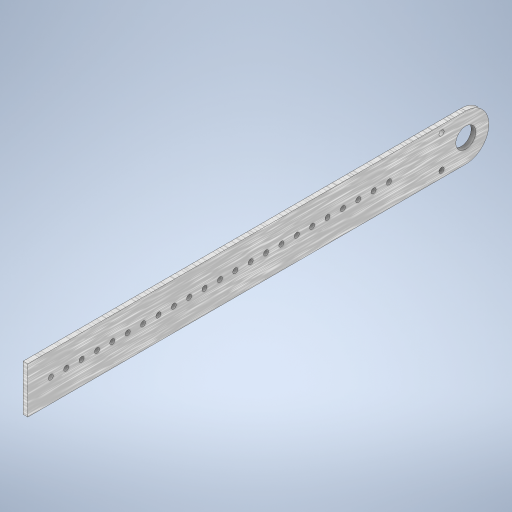
# Autodesk Inventor part: shoulder1_plate_top
Saved by Autodesk Inventor 2024 (Build 280153000, 153)
## iProperties
Company: 細田研究室
Created: 2025-06-07
Part Number: shoulder1_plate_top
Material: アルミニウム 5052
Document SubType Name: Modeling
Designer: HosodaLab2
Density: 2.68 g/cm^3
Appearance: サテン - ブラシ仕上げ 重厚
Mass: 70.367 g
Surface Area: 200.69 cm^2
Volume: 26.0618 cm^3
Stock Number: 1
個数: 1
Author: HosodaLab2
Autodesk Inventor part; units mm, degrees
ref_plane "YZ Plane" through (0, 0, 0) normal (1, 0, 0) x (0, 1, 0)
ref_plane "XZ Plane" through (0, 0, 0) normal (0, 1, 0) x (-1, 0, 0)
ref_plane "XY Plane" through (0, 0, 0) normal (0, 0, 1) x (1, 0, 0)
sketch "スケッチ1" plane through (0, 0, 0) normal (0, 1, 0) x (-1, 0, 0)
  line L0 (0, 0) -> (-300, 0)
  line L1 (-300, 0) -> (-300, -30)
  line L2 (-300, -30) -> (0, -30)
  line L3 (0, -30) -> (0, 0)
  arc A0 (-15, -30) -> (-15, 0) centre (-15, -15) ccw
  point P0 (-15, -15)
  dimension "d0" = 300
  dimension "d1" = 30
  dimension "d2" = 15
  dimension "d3" = 15
  dimension "d43" = 15
  constraints: 8 end point, 2 parallel, 2 point on circle, 2 point on line, 2 tangent, 1 centre point, 1 horizontal, 1 perpendicular
  measures "d0" distance of L2.end L1.end
  measures "d1" distance of L1.end L0.end
  measures "d2" distance from line of L2 point (-15, -15)
  measures "d3" distance from line of point (-15, -15) L3
  measures "d43" distance from line of L3 A0.centre
extrude "押し出し1" add sketch "スケッチ1" along normal blind 3 contours A0 L2 L1 L0
sketch "スケッチ2" plane through (0, 3, 0) normal (0, 1, 0) x (1, 0, 0)
  arc A0 (15, 30) -> (15, 0) centre (15, 15) ccw projected
  line L0 (300, 30) -> (15, 30) projected
  point P0 (0, 0)
  point P1 (15, 15)
  point P2 (0, 15)
  dimension "d6" = 15
  dimension "d7" = 15
  constraints: 1 point on circle
  measures "d6" distance of point (0, 15) point (15, 15)
  measures "d7" distance from line of L0 point (15, 15)
hole "穴1" at (15, 3, -15) direction (0, -1, 0) diameter 13 end through all
sketch "スケッチ3" plane through (0, 3, 0) normal (0, 1, 0) x (1, 0, 0)
  circle A0 centre (15, 15) radius 6.5 projected
  line L0 (15, 15) -> (250, 15)
  line L1 (300, 0) -> (300, 30) projected
  line L2 (250, 15) -> (300, 15)
  point P0 (0, 0)
  point P1 (65, 15)
  point P2 (75, 15)
  point P3 (85, 15)
  point P4 (95, 15)
  point P5 (105, 15)
  point P6 (115, 15)
  point P7 (125, 15)
  point P8 (135, 15)
  point P9 (145, 15)
  point P10 (155, 15)
  point P11 (165, 15)
  point P12 (175, 15)
  point P13 (185, 15)
  point P14 (195, 15)
  point P15 (215, 15)
  point P16 (205, 15)
  point P17 (225, 15)
  point P18 (245, 15)
  point P19 (235, 15)
  point P20 (255, 15)
  point P21 (265, 15)
  point P22 (275, 15)
  point P23 (285, 15)
  point P24 (295, 15)
  dimension "d15" = 50
  dimension "d16" = 10
  dimension "d17" = 10
  dimension "d18" = 10
  dimension "d19" = 10
  dimension "d20" = 10
  dimension "d21" = 10
  dimension "d22" = 10
  dimension "d24" = 10
  dimension "d25" = 10
  dimension "d26" = 10
  dimension "d27" = 10
  dimension "d28" = 10
  dimension "d29" = 10
  dimension "d30" = 10
  dimension "d31" = 10
  dimension "d32" = 10
  dimension "d34" = 10
  dimension "d35" = 10
  dimension "d44" = 10
  dimension "d45" = 10
  dimension "d46" = 10
  dimension "d47" = 10
  dimension "d48" = 10
  constraints: 4 point on line, 3 midpoint, 2 end point, 1 vertical, 22 other
  measures "d15" distance of point (65, 15) A0.centre
  measures "d16" distance of point (65, 15) point (75, 15)
  measures "d17" distance of point (75, 15) point (85, 15)
  measures "d18" distance of point (95, 15) point (85, 15)
  measures "d19" distance of point (95, 15) point (105, 15)
  measures "d20" distance of point (115, 15) point (105, 15)
  measures "d21" distance of point (125, 15) point (115, 15)
  measures "d22" distance of point (125, 15) point (135, 15)
  measures "d24" distance of point (145, 15) point (135, 15)
  measures "d25" distance of point (145, 15) point (155, 15)
  measures "d26" distance of point (155, 15) point (165, 15)
  measures "d27" distance of point (165, 15) point (175, 15)
  measures "d28" distance of point (175, 15) point (185, 15)
  measures "d29" distance of point (185, 15) point (195, 15)
  measures "d30" distance of point (195, 15) point (205, 15)
  measures "d31" distance of point (205, 15) point (215, 15)
  measures "d32" distance of point (215, 15) point (225, 15)
  measures "d34" distance of point (225, 15) point (235, 15)
  measures "d35" distance of point (235, 15) point (245, 15)
  measures "d44" distance of point (245, 15) point (255, 15)
  measures "d45" distance of point (255, 15) point (265, 15)
  measures "d46" distance of point (275, 15) point (265, 15)
  measures "d47" distance of point (275, 15) point (285, 15)
  measures "d48" distance of point (295, 15) point (285, 15)
hole "穴2" at (65, 3, -15) at (75, 3, -15) at (85, 3, -15) at (95, 3, -15) at (105, 3, -15) at (115, 3, -15) at (125, 3, -15) at (135, 3, -15) at (145, 3, -15) at (155, 3, -15) at (165, 3, -15) at (175, 3, -15) at (185, 3, -15) at (195, 3, -15) at (205, 3, -15) at (215, 3, -15) at (225, 3, -15) at (235, 3, -15) at (245, 3, -15) at (255, 3, -15) at (265, 3, -15) at (275, 3, -15) at (285, 3, -15) direction (0, -1, 0) diameter 3.2 end through all
sketch "スケッチ8" plane through (0, 3, 0) normal (0, 1, 0) x (1, 0, 0)
  arc A0 (15, 30) -> (15, 0) centre (15, 15) ccw projected
  line L0 (0, 15) -> (37.6182, 15)
  line L1 (15, 0) -> (300, 0) projected
  circle A1 centre (15, 15) radius 6.5 projected
  point P0 (0, 0)
  point P1 (30.8, 4.5)
  point P2 (30.8, 25.5)
  dimension "d84" = 15
  dimension "d85" = 10.5
  dimension "d86" = 10.5
  dimension "d88" = 15.8
  dimension "d89" = 15.8
  constraints: 2 end point, 1 horizontal, 1 point on circle
  measures "d84" distance between parallel lines of L0 L1
  measures "d85" distance from line of point (30.8, 4.5) L0
  measures "d86" distance from line of point (30.8, 25.5) L0
  measures "d88" horizontal distance of point (30.8, 4.5) A1.centre
  measures "d89" horizontal distance of A1.centre point (30.8, 25.5)
hole "穴6" at (30.8, 3, -4.5) at (30.8, 3, -25.5) direction (0, -1, 0) diameter 3.3 end through all
